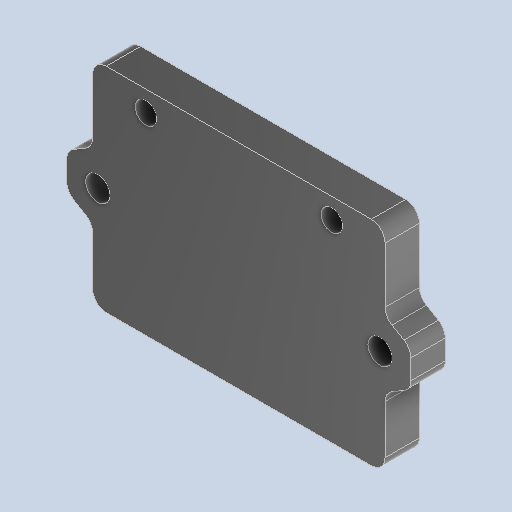
# Autodesk Inventor part: LegBaseBackFrame
Saved by Autodesk Inventor 2024.2 (Build 282272000, 272)
## iProperties
Created: 2024-01-12
Part Number: LegBaseBackFrame
Material: Acetal Resin, Black
Document SubType Name: Modeling
Designer: Masato Kubotera
Density: 1.425 g/cm^3
Appearance: Smooth - Black
Vendor: meviy
Mass: 9.51143 g
Surface Area: 36.2975 cm^2
Volume: 6.67469 cm^3
Author: Masato Kubotera
Autodesk Inventor part; units mm, degrees
ref_plane "YZ Plane" through (0, 0, 0) normal (1, 0, 0) x (0, 1, 0)
ref_plane "XZ Plane" through (0, 0, 0) normal (0, 1, 0) x (-1, 0, 0)
ref_plane "XY Plane" through (0, 0, 0) normal (0, 0, 1) x (1, 0, 0)
derived "LegBaseBackFulcrumFrame.ipt"
sketch "Sketch4" plane through (0, 0, 0) normal (1, 0, 0) x (0, 1, 0)
  circle A0 centre (13.5, 13) radius 1.55 construction
  line L0 (0, 16) -> (21.25, 16)
  line L1 (21.25, 16) -> (21.25, 4.7631)
  line L2 (21.25, 4.7631) -> (25, 2.5981)
  line L3 (25, -2.5981) -> (21.25, -4.7631)
  line L4 (0, 18) -> (0, -27) projected
  line L5 (21.25, 4.7631) -> (25, 2.5981) projected
  line L6 (21.25, -4.7631) -> (25, -2.5981) projected
  line L7 (25, 2.5981) -> (25, -2.5981) projected
  line L8 (17.45, 1.7609) -> (20.5, 3.5218) projected
  arc A1 (21.799, 2.7718) -> (19.201, 2.7718) centre (20.5, 2.0218) ccw projected
  arc A2 (18.749, 2.5109) -> (17.45, 0.2609) centre (18.749, 1.0109) ccw projected
  line L9 (17.45, -1.7609) -> (17.45, 1.7609) projected
  arc A3 (17.45, -0.2609) -> (18.749, -2.5109) centre (18.749, -1.0109) ccw projected
  line L10 (20.5, -3.5218) -> (17.45, -1.7609) projected
  arc A4 (19.201, -2.7718) -> (21.799, -2.7718) centre (20.5, -2.0218) ccw projected
  arc A5 (22.251, -2.5109) -> (23.55, -0.2609) centre (22.251, -1.0109) ccw projected
  line L11 (23.55, -1.7609) -> (20.5, -3.5218) projected
  line L12 (23.55, 1.7609) -> (23.55, -1.7609) projected
  arc A6 (23.55, 0.2609) -> (22.251, 2.5109) centre (22.251, 1.0109) ccw projected
  line L13 (-16.05, 16) -> (16.05, 16) projected
  line L14 (20.5, 3.5218) -> (23.55, 1.7609) projected
  line L15 (21.25, -4.7631) -> (21.25, -15)
  line L16 (21.25, -15) -> (0, -15)
  line L17 (21.25, -15) -> (18, -15) projected
  line L18 (21.25, 27.5) -> (21.25, 4.7631) projected
  point P0 (0, 0)
  point P1 (20.5, 0)
  dimension "d46" = 3.1
  constraints: 12 end point, 5 collinear, 3 point on line, 2 horizontal, 2 vertical, 1 centre point, 1 coincident
  measures "d46" diameter of A0
extrude "Extrusion2" add sketch "Sketch4" along normal blind 5 contours L0 L1 L2 L7 L3 L15 L16 L4 | A2 L8 | L9 A2 | L8 L14 L12 L11 L10 L9 | A1 L8 | L9 A3 | A1 L14 | L10 A3 | A6 L14 | L10 A4 | A6 L12 | L11 A4 | A5 L12 | L11 A5
hole "Hole3" at (0, 20.5, 0) direction (1, 0, 0) diameter 3.5 end through all
hole "Hole4" at (0, 13.5, 13) direction (1, 0, 0) diameter 3.1 end through all
fillet "Fillet1" radius 2 6 edges at (2.5, 21.25, 4.7631) (2.5, 25, 2.5981) (2.5, 25, -2.5981) (2.5, 21.25, -4.7631) (2.5, 21.25, 16) (2.5, 21.25, -15)
mirror "Mirror2" about plane through (0, 0, 0) normal (0, 1, 0)
sketch "Sketch1" plane through (0, 0, 0) normal (1, 0, 0) x (0, 1, 0)
  line L0 (-16, 16) -> (16, 16) construction
  line L1 (16, 16) -> (16, -27) construction
  line L2 (16, -27) -> (-16, -27) construction
  line L3 (-16, -27) -> (-16, 16) construction
  line L4 (-16, 16) -> (16, -27) construction
  line L5 (16, 16) -> (-16, -27) construction
  line L6 (-13.5, 13) -> (13.5, 13) construction
  line L7 (13.5, 13) -> (13.5, -14) construction
  line L8 (13.5, -14) -> (-13.5, -14) construction
  line L9 (-13.5, -14) -> (-13.5, 13) construction
  line L10 (-13.5, 13) -> (13.5, -14) construction
  line L11 (13.5, 13) -> (-13.5, -14) construction
  line L12 (0, 18) -> (0, -27) projected
  circle A0 centre (0, -15) radius 8 construction
  circle A1 centre (0, 0) radius 6 construction
  line L13 (25, 27.5) -> (-25, 27.5) construction
  line L14 (14.2, 11.45) -> (19.3, 11.45) projected
  line L15 (19.3, 11.45) -> (19.3, 18.55) projected
  line L16 (19.3, 18.55) -> (14.2, 11.45) construction
  line L17 (14.2, 18.55) -> (14.2, 11.45) projected
  line L18 (19.3, 18.55) -> (14.2, 18.55) projected
  line L19 (14.2, 18.55) -> (19.3, 11.45) construction
  line L20 (-16.05, -6) -> (-16.05, 16) projected
  line L21 (-16.05, 16) -> (16.05, 16) projected
  line L22 (16.05, 16) -> (16.05, -13.8742) projected
  line L23 (12.25, 27.5) -> (12.25, 18) projected
  line L24 (12.25, 18) -> (-12.25, 18) projected
  line L25 (-12.25, 18) -> (-12.25, 27.5) projected
  arc A2 (19.3, 16.4287) -> (17.1787, 18.55) centre (18.2393, 17.4893) ccw projected
  line L26 (19.3, 15) -> (14.2, 15) construction
  line L27 (16.75, 18.55) -> (16.75, 11.45) construction
  arc A3 (16.3213, 18.55) -> (14.2, 16.4287) centre (15.2607, 17.4893) ccw projected
  arc A4 (17.1787, 11.45) -> (19.3, 13.5713) centre (18.2393, 12.5107) ccw projected
  arc A5 (14.2, 13.5713) -> (16.3213, 11.45) centre (15.2607, 12.5107) ccw projected
  line L28 (17.5, -1.7321) -> (17.5, 1.7321) construction
  line L29 (17.5, 1.7321) -> (20.5, 3.4641) construction
  line L30 (20.5, 3.4641) -> (23.5, 1.7321) construction
  line L31 (23.5, 1.7321) -> (23.5, -1.7321) construction
  line L32 (23.5, -1.7321) -> (20.5, -3.4641) construction
  line L33 (20.5, -3.4641) -> (17.5, -1.7321) construction
  line L34 (-25, 5) -> (19.25, 5) construction
  circle A6 centre (20.5, 0) radius 2.75 construction
  line L35 (16.05, 0) -> (25, 0) construction
  line L36 (20.5, 3.5218) -> (23.55, 1.7609) projected
  line L37 (23.55, 1.7609) -> (23.55, -1.7609) projected
  line L38 (23.55, -1.7609) -> (20.5, -3.5218) projected
  line L39 (20.5, -3.5218) -> (17.45, -1.7609) projected
  line L40 (17.45, -1.7609) -> (17.45, 1.7609) projected
  line L41 (17.45, 1.7609) -> (20.5, 3.5218) projected
  arc A7 (21.799, 2.7718) -> (19.201, 2.7718) centre (20.5, 2.0218) ccw projected
  arc A8 (18.749, 2.5109) -> (17.45, 0.2609) centre (18.749, 1.0109) ccw projected
  arc A9 (17.45, -0.2609) -> (18.749, -2.5109) centre (18.749, -1.0109) ccw projected
  arc A10 (19.201, -2.7718) -> (21.799, -2.7718) centre (20.5, -2.0218) ccw projected
  arc A11 (22.251, -2.5109) -> (23.55, -0.2609) centre (22.251, -1.0109) ccw projected
  arc A12 (23.55, 0.2609) -> (22.251, 2.5109) centre (22.251, 1.0109) ccw projected
  line L42 (21.25, 27.5) -> (21.25, 4.7631) projected
  line L43 (21.25, 4.7631) -> (25, 2.5981) projected
  line L44 (4.5, -7.2058) -> (18, -15) projected
  line L45 (21.25, -4.7631) -> (25, -2.5981) projected
  line L46 (21.25, -4.7631) -> (21.25, -15) projected
  line L47 (21.25, -15) -> (18, -15)
  arc A13 (4.5, -7.2058) -> (0, -6) centre (0, -15) ccw projected
  line L48 (19.25, 18.5) -> (14.25, 18.5) construction
  line L49 (14.25, 18.5) -> (14.25, 11.5) construction
  line L50 (14.25, 11.5) -> (19.25, 11.5) construction
  line L51 (19.25, 11.5) -> (19.25, 18.5) construction
  line L52 (19.25, 18.5) -> (14.25, 11.5) construction
  line L53 (14.25, 18.5) -> (19.25, 11.5) construction
  arc A14 (5.25, -5.9067) -> (3.2786, -5.025) centre (0, -15) ccw projected
  line L54 (5.25, -5.9067) -> (14.25, -11.1029) projected
  line L55 (14.25, -11.1029) -> (14.25, 9.686) projected
  line L56 (0, 0) -> (25, 0) construction
  line L57 (0.75, 14.5) -> (12.7, 14.5) projected
  line L58 (12.7, 14.5) -> (12.7, 14.0737) projected
  arc A15 (12.7, 14.0737) -> (14.25, 9.686) centre (15.2607, 12.5107) ccw projected
  arc A16 (3.2786, -5.025) -> (0.75, 5.9529) centre (0, 0) ccw projected
  line L59 (0.75, 14.5) -> (0.75, 5.9529) projected
  line L60 (25, 2.5981) -> (25, -2.5981) projected
  line L61 (21.25, 27.5) -> (12.25, 27.5) projected
  line L62 (18, -15) -> (21.25, -15) projected
  point P0 (0, -5.5)
  point P1 (0, -0.5)
  point P2 (16.05, -6)
  point P3 (17.45, 1.7609)
  point P4 (17.45, -1.7609)
  point P5 (20.5, -3.5218)
  point P6 (23.55, -1.7609)
  point P7 (23.55, 1.7609)
  point P8 (16.75, 24.5)
  point P9 (16.75, 15)
  point P10 (16.75, 15)
  point P11 (5.9529, -0.75)
  constraints: 2 end point, 3 other
body "Solid2"
